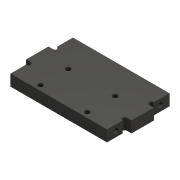
# Autodesk Inventor part: 頭_メインフレームセンター
Saved by Autodesk Inventor 2017.3 (Build 213256000, 256)
## iProperties
Part Number: 頭_メインフレームセンター
Material: アセタール樹脂、黒
Document SubType Name: Modeling
Designer: haya
Mass: 9.25538 g
Surface Area: 33.31 cm^2
Volume: 6.495 cm^3
Density: 1.425 g/cm^3
Appearance: 滑らか - 黒
Author: haya
Autodesk Inventor part; units mm, degrees
ref_plane "YZ Plane" through (0, 0, 0) normal (1, 0, 0) x (0, 1, 0)
ref_plane "XZ Plane" through (0, 0, 0) normal (0, 1, 0) x (-1, 0, 0)
ref_plane "XY Plane" through (0, 0, 0) normal (0, 0, 1) x (1, 0, 0)
sketch "スケッチ1" plane through (0, 0, 0) normal (0, 0, 1) x (1, 0, 0)
  line L0 (0, 0) -> (43.3, 0)
  line L1 (43.3, 28) -> (0, 28)
  line L2 (0, 14) -> (43.3, 14) construction
  line L3 (43.3, 19) -> (45.3, 19)
  line L4 (45.3, 19) -> (45.3, 9)
  line L5 (45.3, 9) -> (43.3, 9)
  arc A0 (43.3, 21) -> (43.3, 19) centre (43.3, 20) ccw
  arc A1 (43.3, 9) -> (43.3, 7) centre (43.3, 8) ccw
  line L6 (43.3, 0) -> (43.3, 7)
  line L7 (43.3, 21) -> (43.3, 28)
  line L8 (21.65, 28) -> (21.65, 0) construction
  line L9 (0, 19) -> (-2, 19)
  line L10 (-2, 19) -> (-2, 9)
  line L11 (-2, 9) -> (0, 9)
  arc A2 (0, 19) -> (0, 21) centre (0, 20) ccw
  arc A3 (0, 7) -> (0, 9) centre (0, 8) ccw
  line L12 (0, 0) -> (0, 7)
  line L13 (0, 21) -> (0, 28)
  dimension "d0" = 43.3
  dimension "d1" = 28
  dimension "d5" = 10
  dimension "d6" = 2
  constraints: 28 end point, 9 symmetric about line, 8 point on circle, 5 perpendicular, 4 centre point, 2 horizontal, 2 midpoint, 2 parallel, 2 point on line, 1 tangent, 5 other
  measures "d0" distance of L0.start L0.end
  measures "d1" distance of L1.end L0.start
  measures "d5" distance of L3.end L4.end
  measures "d6" diameter of A0
extrude "押し出し1" add sketch "スケッチ1" along normal blind 5
sketch "スケッチ3" plane through (43.3, 0, 0) normal (1, 0, 0) x (0, 0, -1)
  line L0 (0, 0) -> (-5, 0) projected
  line L1 (-2.5, 0) -> (-2.5, 28) construction
  line L2 (0, 28) -> (-5, 28) projected
  line L3 (-2.5, 14) -> (0, 14) construction
  line L4 (0, 9) -> (0, 19) projected
  point P0 (-2.5, 24)
  point P1 (-2.5, 4)
  dimension "d7" = 20
  constraints: 4 end point, 4 midpoint, 1 point on line, 1 symmetric about line
  measures "d7" distance of point (-2.5, 4) point (-2.5, 24)
hole "穴1" at (43.3, 24, 2.5) at (43.3, 4, 2.5) direction (-1, 0, 0) diameter 2.4 depth 8 tip angle 118
sketch "スケッチ4" plane through (0, 21, 0) normal (-1, 0, 0) x (0, 0, 1)
  circle A0 centre (2.5, 3) radius 1.2 projected
  circle A1 centre (2.5, -17) radius 1.2 projected
  circle A2 centre (2.5, -17) radius 1.2 projected
  point P0 (0, -21)
hole "穴2" at (0, 24, 2.5) at (0, 4, 2.5) direction (1, 0, 0) diameter 2.4 depth 8 tip angle 118
sketch "スケッチ5" plane through (0, 0, 0) normal (0, 0, -1) x (-1, 0, 0)
  line L0 (0, 0) -> (-43.3, 0) projected
  line L1 (-21.65, 0) -> (-21.65, 28) construction
  line L2 (-43.3, 28) -> (0, 28) projected
  line L3 (-21.65, 8.5) -> (-45.9978, 8.5) construction
  point P0 (-32.15, 2.25)
  point P1 (-11.15, 2.25)
  point P2 (-32.15, 14.75)
  point P3 (-11.15, 14.75)
  dimension "d22" = 21
  dimension "d23" = 12.5
  dimension "d24" = 8.5
  constraints: 4 end point, 3 symmetric about line, 2 midpoint, 1 horizontal, 1 point on line
  measures "d22" distance of point (-32.15, 2.25) point (-11.15, 2.25)
  measures "d23" distance of point (-11.15, 14.75) point (-11.15, 2.25)
  measures "d24" distance between parallel lines of L3 L0
hole "穴3" at (32.15, 2.25, 0) at (11.15, 2.25, 0) at (11.15, 14.75, 0) at (32.15, 14.75, 0) direction (0, 0, 1) diameter 2.1 end through all
